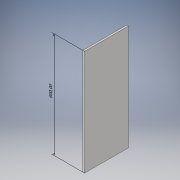
# Autodesk Inventor part: mount_bendPanel
Saved by Autodesk Inventor 2019 (Build 230136000, 136)
## iProperties
Created: 2020-05-22
Part Number: mount_bendPanel
Material: Generic
Document SubType Name: Modeling
Designer: fidg0010a
Density: 1 g/cm^3
Appearance: Default
Author: fidg0010a
Autodesk Inventor part; units mm, degrees
ref_plane "YZ Plane" through (0, 0, 0) normal (1, 0, 0) x (0, 1, 0)
ref_plane "XZ Plane" through (0, 0, 0) normal (0, 1, 0) x (-1, 0, 0)
ref_plane "XY Plane" through (0, 0, 0) normal (0, 0, 1) x (1, 0, 0)
sketch "Sketch4" plane through (0, 0, 0) normal (1, 0, 0) x (0, 1, 0)
  line L0 (450, 125) -> (-150, 125)
  line L1 (-150, 125) -> (-150, 0)
  line L2 (450, 0) -> (450, 125)
  line L3 (450, -125) -> (-150, -125)
  line L4 (-150, -125) -> (-150, 0)
  line L5 (450, 0) -> (450, -125)
  point P0 (0, 0)
  point P1 (0, 0)
  dimension "d3" = 600
  dimension "d5" = 150
  dimension "d9" = 250
  dimension "d10" = 125
  constraints: 12 end point, 3 equal length, 2 coincident, 1 horizontal, 1 perpendicular
  measures "d3" distance between parallel lines of L1 L2
  measures "d5" distance from line of point (0, 0) L1
  measures "d9" distance between parallel lines of L3 L0
  measures "d10" distance from line of point (0, 0) L0
extrude "Extrusion1" add sketch "Sketch4" along normal blind 10
body "Solid1"
